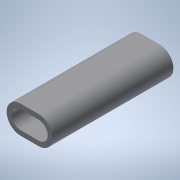
# Autodesk Inventor part: SpectometerTube
Saved by Autodesk Inventor 2020 (Build 240168000, 168)
## iProperties
Created: 2019-09-08
Part Number: SpectometerTube
Material: Polycarbonate, Smoke
Document SubType Name: Modeling
Designer: vmiguel
Density: 1.2 g/cm^3
Appearance: Polycarbonate - Smoked
Author: vmiguel
Autodesk Inventor part; units mm, degrees
ref_plane "YZ Plane" through (0, 0, 0) normal (1, 0, 0) x (0, 1, 0)
ref_plane "XZ Plane" through (0, 0, 0) normal (0, 1, 0) x (-1, 0, 0)
ref_plane "XY Plane" through (0, 0, 0) normal (0, 0, 1) x (1, 0, 0)
sketch "Sketch1" plane through (0, 0, 0) normal (0, 0, 1) x (1, 0, 0)
  line L0 (-15, 0) -> (15, 0) construction
  line L1 (-15, -15) -> (15, -15)
  line L2 (15, 15) -> (-15, 15)
  arc A0 (-15, 15) -> (-15, -15) centre (-15, 0) ccw
  arc A1 (15, -15) -> (15, 15) centre (15, 0) ccw
  line L3 (-15, -23) -> (15, -23)
  arc A2 (15, -23) -> (15, 23) centre (15, 0) ccw
  line L4 (15, 23) -> (-15, 23)
  arc A3 (-15, 23) -> (-15, -23) centre (-15, 0) ccw
  point P0 (0, 0)
  dimension "d0" = 15
  dimension "d1" = 30
  dimension "d2" = 8
  constraints: 12 end point, 8 point on circle, 4 centre point, 4 tangent, 2 parallel, 1 horizontal, 1 midpoint, 3 other
  measures "d0" distance of point (0, 0) L0.end
  measures "d1" diameter of A1
  measures "d2" radial gap between concentric circles of A0 A3
extrude "Extrusion1" add sketch "Sketch1" along normal blind 200
body "Solid1"
